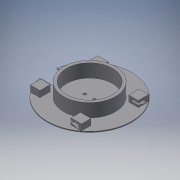
# Autodesk Inventor part: Bauteil1
Saved by Autodesk Inventor 2016 SP2 (Build 200236200, 236)
## iProperties
Created: 2018-09-27
Part Number: Bauteil1
Material: Generisch
Document SubType Name: Modeling
Designer: Nils
Density: 1 g/cm^3
Appearance: Vorgabe
Author: Nils
Autodesk Inventor part; units mm, degrees
ref_plane "YZ Plane" through (0, 0, 0) normal (1, 0, 0) x (0, 1, 0)
ref_plane "XZ Plane" through (0, 0, 0) normal (0, 1, 0) x (-1, 0, 0)
ref_plane "XY Plane" through (0, 0, 0) normal (0, 0, 1) x (1, 0, 0)
sketch "Skizze1" plane through (0, 0, 0) normal (0, 0, 1) x (1, 0, 0)
  circle A0 centre (0, 0) radius 44.5
  line L0 (-31.4663, -31.4663) -> (31.4663, -31.4663) construction
  line L1 (31.4663, -31.4663) -> (31.4663, 31.4663) construction
  line L2 (31.4663, 31.4663) -> (-31.4663, 31.4663) construction
  line L3 (-31.4663, 31.4663) -> (-31.4663, -31.4663) construction
  line L4 (-31.4663, -31.4663) -> (31.4663, 31.4663) construction
  line L5 (31.4663, -31.4663) -> (-31.4663, 31.4663) construction
  line L6 (-26.8774, -27.4663) -> (26.8774, -27.4663)
  line L7 (26.8774, -27.4663) -> (26.8774, -35.4663)
  line L8 (26.8774, -35.4663) -> (-26.8774, -35.4663)
  line L9 (-26.8774, -35.4663) -> (-26.8774, -27.4663)
  line L10 (-26.8774, -27.4663) -> (26.8774, -35.4663) construction
  line L11 (26.8774, -27.4663) -> (-26.8774, -35.4663) construction
  line L12 (-31.4663, -31.4663) -> (31.4663, -31.4663) construction
  line L13 (31.4663, -31.4663) -> (31.4663, 31.4663) construction
  line L14 (31.4663, 31.4663) -> (-31.4663, 31.4663) construction
  line L15 (-31.4663, 31.4663) -> (-31.4663, -31.4663) construction
  line L16 (27.4663, -26.8774) -> (27.4663, 26.8774)
  line L17 (27.4663, 26.8774) -> (35.4663, 26.8774)
  line L18 (35.4663, 26.8774) -> (35.4663, -26.8774)
  line L19 (35.4663, -26.8774) -> (27.4663, -26.8774)
  line L20 (27.4663, -26.8774) -> (35.4663, 26.8774) construction
  line L21 (27.4663, 26.8774) -> (35.4663, -26.8774) construction
  line L22 (31.4663, -31.4663) -> (31.4663, 31.4663) construction
  line L23 (31.4663, 31.4663) -> (-31.4663, 31.4663) construction
  line L24 (-31.4663, 31.4663) -> (-31.4663, -31.4663) construction
  line L25 (-31.4663, -31.4663) -> (31.4663, -31.4663) construction
  line L26 (26.8774, 27.4663) -> (-26.8774, 27.4663)
  line L27 (-26.8774, 27.4663) -> (-26.8774, 35.4663)
  line L28 (-26.8774, 35.4663) -> (26.8774, 35.4663)
  line L29 (26.8774, 35.4663) -> (26.8774, 27.4663)
  line L30 (26.8774, 27.4663) -> (-26.8774, 35.4663) construction
  line L31 (-26.8774, 27.4663) -> (26.8774, 35.4663) construction
  line L32 (31.4663, 31.4663) -> (-31.4663, 31.4663) construction
  line L33 (-31.4663, 31.4663) -> (-31.4663, -31.4663) construction
  line L34 (-31.4663, -31.4663) -> (31.4663, -31.4663) construction
  line L35 (31.4663, -31.4663) -> (31.4663, 31.4663) construction
  line L36 (-27.4663, 26.8774) -> (-27.4663, -26.8774)
  line L37 (-27.4663, -26.8774) -> (-35.4663, -26.8774)
  line L38 (-35.4663, -26.8774) -> (-35.4663, 26.8774)
  line L39 (-35.4663, 26.8774) -> (-27.4663, 26.8774)
  line L40 (-27.4663, 26.8774) -> (-35.4663, -26.8774) construction
  line L41 (-27.4663, -26.8774) -> (-35.4663, 26.8774) construction
  point P0 (0, -31.4663)
  point P1 (31.4663, 0)
  point P2 (0, 31.4663)
  point P3 (-31.4663, 0)
  dimension "d0" = 89
  dimension "d1" = 8
  dimension "d4" = 360
  constraints: 84 end point, 11 midpoint, 4 parallel, 3 perpendicular, 2 horizontal, 2 point on circle, 1 centre point, 1 coincident, 77 other
  measures "d0" diameter of A0
  measures "d1" distance of L6.end L7.end
extrude "Extrusion1" add sketch "Skizze1" along normal blind 10 contours L8 L9 L6 L7
sketch "Skizze2" plane through (0, 0, 0) normal (0, 0, -1) x (-1, 0, 0)
  circle A0 centre (0, 0) radius 44.5
  dimension "d8" = 89
  constraints: 1 centre point, 1 coincident
  measures "d8" diameter of A0
extrude "Extrusion2" add sketch "Skizze2" along normal blind 1
sketch "Skizze3" plane through (-26.8774, -35.4663, 10) normal (0, -1, 0) x (1, 0, 0)
  line L0 (71.3774, -10) -> (-17.6226, -10) construction
  line L1 (51.2372, -10) -> (51.7548, -8.0681) construction
  line L2 (51.7548, -8.0681) -> (2.5176, 5.1249) construction
  line L3 (2.5176, 5.1249) -> (2, 3.1931) construction
  line L4 (2, 3.1931) -> (51.2372, -10) construction
  line L5 (50.3059, -7.6799) -> (50.72, -6.1344) construction
  line L6 (50.72, -6.1344) -> (45.8904, -4.8403) construction
  line L7 (45.8904, -4.8403) -> (45.4763, -6.3858) construction
  line L8 (53.7548, -10) -> (53.7548, 0) construction
  line L9 (0, -10) -> (0, 0) construction
  line L10 (53.7548, -10) -> (0, -10) projected
  line L11 (53.7548, -10) -> (53.7548, 0) projected
  line L12 (0, 0) -> (53.7548, 0) projected
  line L13 (0, -10) -> (0, 0) projected
  line L14 (42.7548, -5.6566) -> (42.7548, -3.5)
  line L15 (42.7548, -3.5) -> (53.7548, -3.5)
  line L16 (53.7548, -10) -> (53.7548, 0) construction
  line L17 (42.7548, -7.7272) -> (42.7548, -10)
  line L18 (53.7548, -10) -> (0, -10) construction
  line L19 (53.7548, -10) -> (0, -10) projected
  line L20 (42.7548, -10) -> (53.7548, -10)
  line L21 (53.7548, -10) -> (53.7548, -3.5)
  line L22 (42.7548, -5.6566) -> (45.4763, -6.3858)
  line L23 (45.4763, -6.3858) -> (45.8904, -4.8403)
  line L24 (45.8904, -4.8403) -> (50.72, -6.1344)
  line L25 (50.72, -6.1344) -> (50.3059, -7.6799)
  line L26 (50.3059, -7.6799) -> (51.7548, -8.0681)
  line L27 (51.2372, -10) -> (51.7548, -8.0681)
  line L28 (51.2372, -10) -> (42.7548, -7.7272)
  line L29 (0, -10) -> (0, 0) projected
  line L30 (42.7548, -10) -> (0, -10)
  line L31 (53.7548, -3.5) -> (53.7548, 0)
  line L32 (53.7548, 0) -> (0, 0) projected
  line L33 (0, -10) -> (0, 0)
  line L34 (0, 0) -> (53.7548, 0)
  line L35 (53.7548, -3.5) -> (53.7548, 0)
  line L36 (53.7548, 0) -> (0, 0)
  line L37 (0, 0) -> (0, -10)
  line L38 (0, -10) -> (42.7548, -10)
  line L39 (42.7548, -10) -> (42.7548, -7.7272)
  line L40 (42.7548, -7.7272) -> (51.2372, -10)
  line L41 (51.2372, -10) -> (51.7548, -8.0681)
  line L42 (51.7548, -8.0681) -> (50.3059, -7.6799)
  line L43 (42.7548, -5.6566) -> (42.7548, -3.5)
  line L44 (42.7548, -3.5) -> (53.7548, -3.5)
  point P0 (26.8774, -10)
  dimension "d11" = 2
  dimension "d12" = 1.6
  dimension "d13" = 15
  dimension "d14" = 1.5
  dimension "d15" = 2
  dimension "d16" = 2
  dimension "d17" = 5
  dimension "d18" = 50.9741
  dimension "d19" = 11
  dimension "d20" = 6.5
  dimension "d36" = 15.1249
  dimension "d37" = 8.6249
  constraints: 66 end point, 16 collinear, 11 perpendicular, 7 point on line, 3 parallel, 2 vertical, 1 horizontal
  measures "d11" distance of L2.end L3.end
  measures "d12" distance of L5.start L5.end
  measures "d13" angle of L4 L0
  measures "d14" distance between parallel lines of L1 L5
  measures "d15" distance from line of L8 L1.end
  measures "d16" distance from line of L3.end L9
  measures "d17" distance of L5.end L6.end
  measures "d18" distance of L1.end L2.end
  measures "d19" distance of L14.end L15.end
  measures "d20" distance between parallel lines of L0 L15
  measures "d36" distance from line of L2.end L0
  measures "d37" distance from line of L2.end L15
extrude "Extrusion3" cut sketch "Skizze3" against normal blind 8 contours L28 L17 L10 L13 L12 L11 L15 L14 L22 L23 L24 L25 L26 L27
sketch "Skizze4" plane through (15.8774, -27.4663, 6.5) normal (0, 1, 0) x (1, 0, 0)
  line L0 (11, 6.5) -> (11, 0) projected
  line L1 (-60.3774, 6.5) -> (28.6226, 6.5) projected
  line L2 (11, 0) -> (0, 0)
  line L3 (0, 0) -> (0, 6.5)
  line L4 (0, 6.5) -> (11, 6.5)
  line L5 (11, 6.5) -> (11, 0)
  line L6 (0, 6.5) -> (0, 4.2272) projected
  point P0 (-15.8774, 6.5)
  constraints: 8 end point, 2 parallel, 1 horizontal, 1 perpendicular
extrude "Extrusion4" add sketch "Skizze4" along normal blind 2
pattern_circular "Runde Anordnung1" count 4 over 360 about axis through (0, 0, 0) along (0, 0, -1) of "Extrusion1", "Extrusion3", "Extrusion4"
sketch "Skizze5" plane through (0, 0, 0) normal (0, 0, 1) x (1, 0, 0)
  line L0 (-27.4663, -27.4663) -> (27.4663, -27.4663) construction
  line L1 (27.4663, -27.4663) -> (27.4663, 27.4663) construction
  line L2 (27.4663, 27.4663) -> (-27.4663, 27.4663) construction
  line L3 (-27.4663, 27.4663) -> (-27.4663, -27.4663) construction
  line L4 (-25.4663, -15.8774) -> (-25.4663, -26.8774) construction
  line L5 (15.8774, -25.4663) -> (26.8774, -25.4663) construction
  line L6 (25.4663, 15.8774) -> (25.4663, 26.8774) construction
  line L7 (-15.8774, 25.4663) -> (-26.8774, 25.4663) construction
  circle A0 centre (0, 0) radius 27.25
  circle A1 centre (0, 0) radius 24.25
  dimension "d28" = 2
  dimension "d29" = 2
  dimension "d30" = 2
  dimension "d31" = 2
  dimension "d32" = 54.5
  dimension "d33" = 3
  constraints: 8 end point, 2 centre point, 2 parallel, 1 coincident, 1 horizontal, 1 perpendicular
  measures "d28" distance between parallel lines of L4 L3
  measures "d29" distance between parallel lines of L5 L0
  measures "d30" distance between parallel lines of L6 L1
  measures "d31" distance between parallel lines of L7 L2
  measures "d32" diameter of A0
  measures "d33" radial gap between concentric circles of A0 A1
extrude "Extrusion5" add sketch "Skizze5" along normal blind 14
sketch "Skizze6" plane through (0, 0, 0) normal (0, 0, 1) x (1, 0, 0)
  line L0 (-35.35, -9) -> (-44.0908, -9) projected
  line L1 (-44.0908, 9) -> (-35.35, 9) projected
  line L2 (-35.35, -9) -> (-35.35, 9) construction
  arc A0 (-26.8774, 35.4663) -> (-35.4663, -26.8774) centre (0, 0) ccw projected
  arc A1 (-43.5804, 9) -> (-43.5804, -9) centre (0, 0) ccw
  line L3 (-43.5804, 9) -> (-35.35, 9)
  line L4 (-43.5804, -9) -> (-35.35, -9)
  line L5 (-35.35, -9) -> (-27.5709, -9)
  line L6 (-27.5709, -9) -> (-27.5709, 9)
  line L7 (-27.5709, 9) -> (-35.35, 9)
  constraints: 12 end point, 4 point on circle, 2 collinear, 2 perpendicular, 2 point on line, 1 centre point, 1 horizontal, 1 vertical
extrude "Extrusion6" cut sketch "Skizze6" against normal blind 1
sketch "Skizze7" plane through (0, 0, 0) normal (0, 0, 1) x (1, 0, 0)
  line L0 (0, 0) -> (-5, 0)
  circle A0 centre (-5, 0) radius 1.5
  line L1 (0, 0) -> (5, 0)
  circle A1 centre (5, 0) radius 1.5
  dimension "d40" = 5
  dimension "d41" = 3
  dimension "d42" = 5
  dimension "d43" = 3
  constraints: 4 end point, 2 centre point, 2 coincident, 2 horizontal
  measures "d40" distance of L0.start L0.end
  measures "d41" diameter of A0
  measures "d42" distance of L0.start L1.end
  measures "d43" diameter of A1
extrude "Extrusion7" cut sketch "Skizze7" against normal blind 10
equation "\"d42\" = d40"
